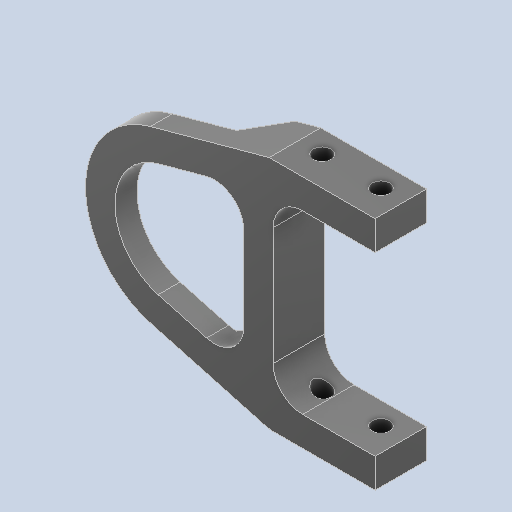
# Autodesk Inventor part: Lower Guide
Saved by Autodesk Inventor 2024 (Build 280153000, 153)
## iProperties
Created: 2023-12-21
Part Number: Lower Guide
Material: Generic
Document SubType Name: Modeling
Designer: greg
Density: 1 g/cm^3
Appearance: Smooth - Black
Author: greg
## iProperties of the stored document Lower Guide_3DPrint.ipt
Created: 2023-12-21
Part Number: Lower Guide_3DPrint
Material: Generic
Document SubType Name: Modeling
Designer: greg
Density: 1 g/cm^3
Appearance: Default
Author: greg
Autodesk Inventor part; units mm, degrees
ref_plane "YZ Plane" through (0, 0, 0) normal (1, 0, 0) x (0, 1, 0)
ref_plane "XZ Plane" through (0, 0, 0) normal (0, 1, 0) x (-1, 0, 0)
ref_plane "XY Plane" through (0, 0, 0) normal (0, 0, 1) x (1, 0, 0)
sketch "Sketch2" plane through (0, 0, 0) normal (0, 0, 1) x (1, 0, 0)
  arc A0 (-42.61997, 14.00175) -> (-42.61997, 42.89425) centre (-44.7675, 28.448) ccw
  line L0 (-19.05, 53.848) -> (-6.35, 53.848)
  line L1 (-6.35, 3.048) -> (-19.05, 3.048)
  line L2 (-8.255, 3.048) -> (-4.445, 3.048)
  line L3 (-20.955, 3.048) -> (-17.145, 3.048)
  line L4 (-4.445, 53.848) -> (-8.255, 53.848)
  line L5 (-17.145, 53.848) -> (-20.955, 53.848)
  circle A1 centre (-44.7675, 28.448) radius 12.7
  arc A2 (-49.797098, 46.822048) -> (-49.797098, 10.073952) centre (-44.7675, 28.448) ccw
  line L6 (-24.13, 3.048) -> (-49.797098, 10.073952)
  line L7 (-49.797098, 46.822048) -> (-24.13, 53.848)
  line L8 (-1.27, 3.048) -> (-1.27, 9.398)
  line L9 (-1.27, 53.848) -> (-1.27, 47.498)
  line L10 (-1.27, 9.398) -> (-23.276593, 9.398)
  line L11 (-23.276593, 9.398) -> (-48.120565, 16.198635)
  line L12 (-48.120565, 40.697365) -> (-23.276593, 47.498)
  line L13 (-23.276593, 47.498) -> (-1.27, 47.498)
  line L14 (-1.27, 3.048) -> (-24.13, 3.048)
  line L15 (-24.13, 53.848) -> (-1.27, 53.848)
  line L16 (-23.276593, 9.398) -> (-23.276593, 47.498)
  line L17 (-29.626593, 11.13621) -> (-29.626593, 45.75979)
  point P0 (0, 0)
  point P1 (-12.7, 3.048)
  point P2 (-12.7, 53.848)
extrude "Extrusion1" add sketch "Sketch2" against normal blind 4.7625 contours L11 L10 L8 L14 L2 L1 L3 L6 A2 L7 L15 L5 L0 L4 L9 L13 L12 A1 | L17 L12 L16 L11
fillet "Fillet1" radius 6.35 4 edges at (-29.6266, 11.1362, -2.3813) (-29.6266, 45.7598, -2.3813) (-23.2766, 47.498, -2.3813) (-23.2766, 9.398, -2.3813)
sketch "Sketch3" plane through (0, 0, -4.7625) normal (0, 0, -1) x (-1, 0, 0)
  line L0 (1.27, 47.498) -> (16.926593, 47.498)
  arc A0 (23.276593, 41.148) -> (16.926593, 47.498) centre (16.926593, 41.148) ccw
  line L1 (23.276593, 41.148) -> (23.276593, 15.748)
  arc A1 (16.926593, 9.398) -> (23.276593, 15.748) centre (16.926593, 15.748) ccw
  line L2 (16.926593, 9.398) -> (1.27, 9.398)
  line L3 (1.27, 9.398) -> (1.27, 3.048)
  line L4 (1.27, 3.048) -> (24.13, 3.048)
  line L5 (24.13, 3.048) -> (49.797098, 10.073952)
  arc A2 (49.797098, 10.073952) -> (49.797098, 46.822048) centre (44.7675, 28.448) ccw
  line L6 (49.797098, 46.822048) -> (24.13, 53.848)
  line L7 (24.13, 53.848) -> (1.27, 53.848)
  line L8 (1.27, 53.848) -> (1.27, 47.498)
  line L9 (48.120565, 16.198635) -> (37.653126, 13.333343)
  arc A3 (29.626593, 19.458025) -> (37.653126, 13.333343) centre (35.976593, 19.458025) ccw
  line L10 (29.626593, 19.458025) -> (29.626593, 37.437975)
  arc A4 (37.653126, 43.562657) -> (29.626593, 37.437975) centre (35.976593, 37.437975) ccw
  line L11 (37.653126, 43.562657) -> (48.120565, 40.697365)
  arc A5 (48.120565, 16.198635) -> (48.120565, 40.697365) centre (44.7675, 28.448) ccw
  line L12 (29.626593, 19.458025) -> (29.626593, 4.552603)
  line L13 (29.626593, 37.437975) -> (29.626593, 52.343397)
  point P0 (0, 0)
  constraints: 4 end point, 3 point on line, 1 vertical
extrude "Extrusion2" add sketch "Sketch3" along normal blind 6.35 contours L8 L7 L6 L13 L10 L12 L5 L4 L3 L2 A1 L1 A0 L0
chamfer "Chamfer1" distance 6.35 angle 45 2 edges at (-29.6266, 44.8907, -4.7625) (-29.6266, 12.0053, -4.7625)
sketch "Sketch4" plane through (-24.13, 3.048, 0) normal (0, -1, 0) x (1, 0, 0)
  circle A0 centre (17.78, -6.35) radius 1.905 projected
  circle A1 centre (5.08, -6.35) radius 1.905 projected
  point P0 (24.13, 0)
extrude "Extrusion3" cut sketch "Sketch4" against normal through all
body "Solid1"
